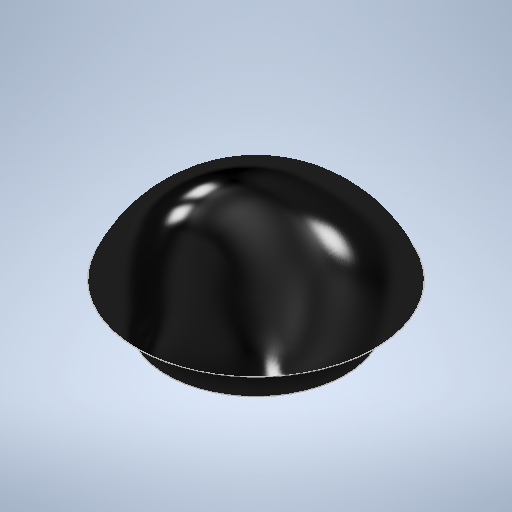
# Autodesk Inventor part: Hephaestus38v2 Case Feet
Saved by Autodesk Inventor 2025 (Build 290162000, 162)
## iProperties
Created: 2025-12-13
Part Number: Hephaestus38v2 Case Feet
Material: Thermoplastic Resin
Document SubType Name: Modeling
Designer: User
Density: 1.28 g/cm^3
Appearance: Black
Author: User
Autodesk Inventor part; units mm, degrees
ref_plane "YZ Plane" through (0, 0, 0) normal (1, 0, 0) x (0, 1, 0)
ref_plane "XZ Plane" through (0, 0, 0) normal (0, 1, 0) x (-1, 0, 0)
ref_plane "XY Plane" through (0, 0, 0) normal (0, 0, 1) x (1, 0, 0)
sketch "Sketch1" plane through (0, 0, 0) normal (0, 1, 0) x (-1, 0, 0)
  circle A0 centre (0, 0) radius 2.25
  circle A1 centre (0, 0) radius 1.9
  dimension "d0" = 4.5
  dimension "d1" = 3.8
  constraints: 2 centre point, 2 coincident
  measures "d0" diameter of A0
  measures "d1" diameter of A1
extrude "Extrusion1" add sketch "Sketch1" along normal blind 0.96
sketch "Sketch2" plane through (0, 0, 0) normal (1, 0, 0) x (0, 1, 0)
  arc A0 (0.96, -3) -> (0.96, 3) centre (-0.29, 0) ccw
  line L0 (0.96, -2.25) -> (0.96, 2.25) projected
  line L1 (0.96, 3) -> (0.96, 2.25)
  line L2 (0.96, -3) -> (0.96, -2.25)
  line L3 (2.96, 0) -> (0.96, 0)
  point P0 (0, 0)
  dimension "d4" = 2
  dimension "d5" = 3
  constraints: 6 end point, 3 collinear, 3 point on circle, 1 centre point, 1 midpoint
  measures "d4" distance edge to line of A0 L0
  measures "d5" distance from line of L3 L1.start
revolve "Revolution1" add sketch "Sketch2" angle 360 about axis through (0, 2.96, 0) along (0, -1, 0) contours L3 L0 L1 A0
sketch "Sketch3" plane through (0, 0.96, 0) normal (0, -1, 0) x (1, 0, 0)
  line L0 (-2.25, 1) -> (2.25, 1)
  line L1 (2.25, 1) -> (2.25, -1)
  line L2 (2.25, -1) -> (-2.25, -1)
  line L3 (-2.25, -1) -> (-2.25, 1)
  line L4 (-2.25, 1) -> (2.25, -1) construction
  line L5 (2.25, 1) -> (-2.25, -1) construction
  circle A0 centre (0, 0) radius 2.25 projected
  circle A1 centre (0, 0) radius 1.9 projected
  point P0 (1.6155, 1)
  point P1 (-1.6155, 1)
  point P2 (-1.6155, -1)
  point P3 (1.6155, -1)
  dimension "d7" = 2
  constraints: 12 end point, 2 midpoint, 2 parallel, 1 horizontal, 1 perpendicular, 1 tangent
  measures "d7" distance between parallel lines of L2 L0
extrude "Extrusion2" cut sketch "Sketch3" against normal blind 0.16 contours L0 A1 L2
body "Solid1"
